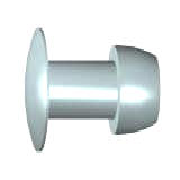
# Autodesk Inventor part: IFI 114 - .125  x .36
Saved by Autodesk Inventor 2012 (Build 160160000, 160)
## iProperties
Created: 2011-02-07
Part Number: IFI 114 - .125  x .36
Material: Steel, Mild
Description: Regular Protruding Head Style Break Mandrel Blind Rivet - Inch
Document SubType Name: Modeling
Standard: IFI 114
Designer: t_walti
Standard Revision: 2003
Standards Organization: ANSI
Language: en-US
Size Designation: 66
Categories: <MemberInstance><Categories><Category DisplayName="Fasteners" InternalName="e4da775c-781d-43d5-af7c-5136215cf5a6" Mnemonic="FSTN"><Category DisplayName="Rivets" InternalName="cf3d8c00-4198-4f00-854b-0d52b0adb238" Mnemonic="RIVET"><CategoryParameter DisplayName="Nominal Diameter" InternalName="0b221833-a430-4b2f-a4d4-a4e7cdbab5fe" Mnemonic="nomdia"/><CategoryParameter DisplayName="Nominal Length" InternalName="184b63f4-60b5-4ddb-b59d-a876aedee7db" Mnemonic="nomlen"/><CategoryParameter DisplayName="Functional Length" InternalName="2e4ddd0b-69f7-4d63-b45a-ef59153ff940" Mnemonic="fnclen"/><CategoryParameter DisplayName="Type" InternalName="841ce55c-7089-4646-bdbb-4888c77f269c" Mnemonic="type"/><CategoryParameter DisplayName="Grip Range (Min.-Max.)" InternalName="b095e0a4-6026-43f1-9b5f-1a93f7499cb0" Mnemonic="grprng"/><Category DisplayName="Plain" InternalName="0955f08f-2c95-4108-bac3-e7e722525866" Mnemonic="PLNRIVET"/></Category></Category><Category DisplayName="DataType" InternalName="23b78d0f-2648-40c6-8793-ca6db495c9e8" Mnemonic="DATATYPE"><CategoryParameter DisplayName="DisplayName" InternalName="05415f3d-3907-474b-a020-eb9d644f4cf3" Mnemonic="DISPLAYNAME"/><CategoryParameter DisplayName="InternalName" InternalName="cf1d0246-76d9-4b4a-8305-fa0409afb5c1" Mnemonic="INTERNALNAME"/><CategoryParameter DisplayName="Folder Name" InternalName="3f06958e-8713-4116-9be7-ed6184ecc97b" Mnemonic="FOLDERNAME"/><CategoryParameter DisplayName="Family Version" InternalName="914462f6-6e19-4b14-ba84-155b9680b1d0" Mnemonic="FAMILYREVISION"/><CategoryParameter DisplayName="ClipFormat" InternalName="bc51e27b-3422-4e78-93ef-cec197ddf230" Mnemonic="CLIPFORMAT"/><CategoryParameter DisplayName="IsMetric" InternalName="e2385c5b-1ea4-4823-96a8-8de651266ec3" Mnemonic="ISMETRIC"/><CategoryParameter DisplayName="Description" InternalName="13903e3d-64b1-4950-80da-f627842ea37f" Mnemonic="DESCRIPTION"/><CategoryParameter DisplayName="StdsOrg" InternalName="8f5914e1-4693-403f-8ab5-d37768198c9d" Mnemonic="STDSORG"/><CategoryParameter DisplayName="Standard" InternalName="0c0a119c-1e12-4c84-803f-101930972f5e" Mnemonic="STANDARD"/><CategoryParameter DisplayName="Manufacturer" InternalName="cd6c7a72-a28a-4e50-99a9-2c7f4e13e5ad" Mnemonic="MANUFACTURER"/><CategoryParameter DisplayName="Member Revision" InternalName="a65d44b9-392f-4f4f-857b-e4b3d54996fe" Mnemonic="MEMBERREVISION"/><CategoryParameter DisplayName="Standard Revision" InternalName="91d5a463-65c2-4fde-b823-3b7fea5e8e17" Mnemonic="STANDARDREVISION"/><CategoryParameter DisplayName="Revision Guid" InternalName="45a75005-10b1-4dfc-8d6d-dfe629f0b93c" Mnemonic="REVISIONGUID"/><CategoryParameter DisplayName="Designation" InternalName="2675968c-4ce5-49e0-a4f5-552d29089031" Mnemonic="DESIGNATION"/><CategoryParameter DisplayName="FileName" InternalName="8b46a4cc-9585-4fed-90c3-899f57e09a73" Mnemonic="FILENAME"/><CategoryParameter DisplayName="Default Row" InternalName="2af9ec52-faaa-4026-b378-f9fa4afca842" Mnemonic="DEFAULTROW"/><Category DisplayName="Part" InternalName="c0e0b642-3bcb-4cc8-9e80-f96d35c4afa4" Mnemonic="PART"><CategoryParameter DisplayName="Material" InternalName="818a152a-d3c3-49ca-80ee-df7d91421b8e" Mnemonic="MATERIAL"/><CategoryParameter DisplayName="Material Key" InternalName="5c9a8adb-dd2b-4535-b97f-0a94a95fe41f" Mnemonic="MATERIALKEY"/><CategoryParameter DisplayName="Part Number" InternalName="016b6077-bfbe-49bd-92c9-d8d59c39c941" Mnemonic="PARTNUMBER"/><CategoryParameter DisplayName="Stock Number" InternalName="4dba7c1c-e26c-444e-836c-b08b433409a8" Mnemonic="STOCKNUMBER"/></Category></Category><Category DisplayName="LegacyMap" InternalName="cd87c42b-3e48-431e-b5c0-1cbeb14dfe77" Mnemonic="LEGACYMAP"><CategoryParameter DisplayName="CatalogName" InternalName="d99d1e27-aa94-4de2-af4c-c348882a6f4f" Mnemonic="CATALOGNAME"/><CategoryParameter DisplayName="FamilyNumber" InternalName="e705e1f4-09cb-413e-91f9-551b4188271e" Mnemonic="FAMILYNUMBER"/><CategoryParameter DisplayName="MemberID" InternalName="8e5e0294-fc51-4c8f-b3d7-003dc5ed94f6" Mnemonic="MEMBERID"/><CategoryParameter DisplayName="unique CC member ID" InternalName="5193edd4-b2b0-4ab4-9d54-de900eee34e0" Mnemonic="CCCOOKIE"/><CategoryParameter DisplayName="unique DA member ID" InternalName="0918ad47-427f-4fed-ae26-24c81c58f590" Mnemonic="DACOOKIE"/><CategoryParameter DisplayName="Merge11 ID" InternalName="0ee8fb18-e2ed-4f39-96f6-1f4b5f50aa71" Mnemonic="MERGE11"/><CategoryParameter DisplayName="Split ID" InternalName="72b5c83c-be7f-45c4-ae51-9160ea6deb26" Mnemonic="SPLIT"/></Category></Categories><FamilyTemplate Id="ri0001"><FamilyTemplateParameters><FamilyTemplateParameter ObjectType="kUserParameterObject" ValueType="xs:double" Id="1" ObjectReferenceKey="R1"/><FamilyTemplateParameter ObjectType="kUserParameterObject" ValueType="xs:double" Id="2" ObjectReferenceKey="KOD"/><FamilyTemplateParameter ObjectType="kUserParameterObject" ValueType="xs:double" Id="3" ObjectReferenceKey="BOR"/><FamilyTemplateParameter ObjectType="kUserParameterObject" ValueType="xs:double" Id="4" ObjectReferenceKey="PHH"/><FamilyTemplateParameter ObjectType="kUserParameterObject" ValueType="xs:double" Id="5" ObjectReferenceKey="NND"/><FamilyTemplateParameter ObjectType="kUserParameterObject" ValueType="xs:double" Id="6" ObjectReferenceKey="KLG"/><FamilyTemplateParameter ObjectType="kUserParameterObject" ValueType="xs:double" Id="7" ObjectReferenceKey="KLGMAX"/><FamilyTemplateParameter ObjectType="kUserParameterObject" ValueType="xs:double" Id="8" ObjectReferenceKey="KOH"/><FamilyTemplateParameter ObjectType="kUserParameterObject" ValueType="xs:double" Id="9" ObjectReferenceKey="KLGMIN"/><FamilyTemplateParameter ObjectType="kPropertyObject" ValueType="xs:string" Id="100" ObjectReferenceKey="{32853F0F-3444-11d1-9E93-0060B03C1CA6}" SubObjectId="52"/><FamilyTemplateParameter ObjectType="kPropertyObject" ValueType="xs:string" Id="105" ObjectReferenceKey="{32853F0F-3444-11d1-9E93-0060B03C1CA6}" SubObjectId="5"/><FamilyTemplateParameter ObjectType="kPartComponentDefinitionObject" ValueType="xs:string" Id="110" SubObjectId="Material"/></FamilyTemplateParameters></FamilyTemplate><CategoryParameterMap><ParamToTemplateMap><ParamToTemplate CategoryParameter="//CategoryParameter[@InternalName='05415f3d-3907-474b-a020-eb9d644f4cf3']" ConstantValue="Regular Protruding Head Style Break Mandrel Blind Rivet (Inch) (IFI)"/><ParamToTemplate CategoryParameter="//CategoryParameter[@InternalName='cf1d0246-76d9-4b4a-8305-fa0409afb5c1']" ConstantValue="b007ff4d-50a3-4cbc-aa5a-b75e20d450cd"/><ParamToTemplate CategoryParameter="//CategoryParameter[@InternalName='3f06958e-8713-4116-9be7-ed6184ecc97b']" ConstantValue="IFI 114(4)"/><ParamToTemplate CategoryParameter="//CategoryParameter[@InternalName='914462f6-6e19-4b14-ba84-155b9680b1d0']" ConstantValue="10"/><ParamToTemplate CategoryParameter="//CategoryParameter[@InternalName='bc51e27b-3422-4e78-93ef-cec197ddf230']" ConstantValue="CF_INVENTOR.STDPARTS"/><ParamToTemplate CategoryParameter="//CategoryParameter[@InternalName='e2385c5b-1ea4-4823-96a8-8de651266ec3']" ConstantValue="false"/><ParamToTemplate CategoryParameter="//CategoryParameter[@InternalName='13903e3d-64b1-4950-80da-f627842ea37f']" ConstantValue="Regular Protruding Head Style Break Mandrel Blind Rivet - Inch"/><ParamToTemplate CategoryParameter="//CategoryParameter[@InternalName='8f5914e1-4693-403f-8ab5-d37768198c9d']" ConstantValue="ANSI"/><ParamToTemplate CategoryParameter="//CategoryParameter[@InternalName='0c0a119c-1e12-4c84-803f-101930972f5e']" ConstantValue="IFI 114"/><ParamToTemplate CategoryParameter="//CategoryParameter[@InternalName='cd6c7a72-a28a-4e50-99a9-2c7f4e13e5ad']" TemplateParameter="104"/><ParamToTemplate CategoryParameter="//CategoryParameter[@InternalName='91d5a463-65c2-4fde-b823-3b7fea5e8e17']" ConstantValue="2003"/><ParamToTemplate CategoryParameter="//CategoryParameter[@InternalName='45a75005-10b1-4dfc-8d6d-dfe629f0b93c']" ConstantValue="92a414c9-0dfd-4a8a-86e0-b3adb112cc1b"/><ParamToTemplate CategoryParameter="//CategoryParameter[@InternalName='2af9ec52-faaa-4026-b378-f9fa4afca842']" ConstantValue="10"/><ParamToTemplate CategoryParameter="//CategoryParameter[@InternalName='d99d1e27-aa94-4de2-af4c-c348882a6f4f']" ConstantValue="ANSI"/><ParamToTemplate CategoryParameter="//CategoryParameter[@InternalName='e705e1f4-09cb-413e-91f9-551b4188271e']" ConstantValue="1123"/><ParamToTemplate CategoryParameter="//CategoryParameter[@InternalName='8b46a4cc-9585-4fed-90c3-899f57e09a73']" ConstantValue="IFI 114 - 66 x .36(4)"/><ParamToTemplate CategoryParameter="//CategoryParameter[@InternalName='a65d44b9-392f-4f4f-857b-e4b3d54996fe']" ConstantValue="c1e365bb-b061-42a6-b7ff-1cacd618005e"/><ParamToTemplate CategoryParameter="//CategoryParameter[@InternalName='184b63f4-60b5-4ddb-b59d-a876aedee7db']" ConstantValue="0.575"/><ParamToTemplate CategoryParameter="//CategoryParameter[@InternalName='b095e0a4-6026-43f1-9b5f-1a93f7499cb0']" ConstantValue="0.251 - 0.375"/><ParamToTemplate CategoryParameter="//CategoryParameter[@InternalName='8e5e0294-fc51-4c8f-b3d7-003dc5ed94f6']" ConstantValue="210"/><ParamToTemplate CategoryParameter="//CategoryParameter[@InternalName='2675968c-4ce5-49e0-a4f5-552d29089031']" TemplateParameter="100"/><ParamToTemplate CategoryParameter="//CategoryParameter[@InternalName='2e4ddd0b-69f7-4d63-b45a-ef59153ff940']" TemplateParameter="6"/><ParamToTemplate CategoryParameter="//CategoryParameter[@InternalName='818a152a-d3c3-49ca-80ee-df7d91421b8e']" TemplateParameter="110"/><ParamToTemplate CategoryParameter="//CategoryParameter[@InternalName='0b221833-a430-4b2f-a4d4-a4e7cdbab5fe']" TemplateParameter="5"/><ParamToTemplate CategoryParameter="//CategoryParameter[@InternalName='016b6077-bfbe-49bd-92c9-d8d59c39c941']" TemplateParameter="105"/></ParamToTemplateMap></CategoryParameterMap></MemberInstance>
Density: 7.86 g/cm^3
Mass: 1.48656 g
Surface Area: 2.5312 cm^2
Volume: 0.18913 cm^3
IsCustomPart: 1
Author: t_walti
Autodesk Inventor part; units mm, degrees
ref_plane "YZ Plane" through (0, 0, 0) normal (1, 0, 0) x (0, 1, 0)
ref_plane "XZ Plane" through (0, 0, 0) normal (0, 1, 0) x (-1, 0, 0)
ref_plane "XY Plane" through (0, 0, 0) normal (0, 0, 1) x (1, 0, 0)
sketch "Sketch1" plane through (0, 0, 0) normal (0, 0, 1) x (1, 0, 0)
  line L0 (-0.2794, 3.3401) -> (0, 3.3401)
  line L1 (0, 3.3401) -> (0, 1.5875)
  line L2 (0, 1.5875) -> (9.145, 1.5875)
  line L3 (9.145, 1.5875) -> (9.145, 2.4049)
  line L4 (-1.524, 0) -> (13.717, 0)
  arc A0 (-0.2794, 3.3401) -> (-1.524, 0) centre (3.5802, 0) ccw
  line L5 (13.717, 0) -> (13.717, 1.8371)
  arc A1 (13.717, 1.8371) -> (9.145, 2.4049) centre (10.6582, -4.1017) ccw
  line L6 (-4.95, 0) -> (16.8866, 0) projected
  line L7 (0, -8.6865) -> (0, 7.3745) projected
  dimension "d0" = 6.6802
  dimension "d1" = 3.175
  dimension "d2" = 4.8097
  dimension "d3" = 3.6741
  dimension "d4" = 6.6802
  dimension "d5" = 4.572
  dimension "d6" = 9.145
  dimension "d7" = 0.2794
  dimension "d8" = 1.524
  constraints: 12 end point, 4 point on circle, 3 perpendicular, 2 centre point, 2 collinear, 2 parallel, 1 horizontal, 1 point on line
  measures "d0" diameter of L0 L4
  measures "d1" diameter of L2 L4
  measures "d2" diameter of L3.end L4
  measures "d3" diameter of L5.end L4
  measures "d4" radius of A1
  measures "d5" distance between parallel lines of L5 L3
  measures "d6" distance of L1.end L2.end
  measures "d7" distance of L0.start L0.end
  measures "d8" distance from line of L4.start L1
revolve "Body" add sketch "Sketch1" angle 360 about axis through (-1.524, 0, 0) along (1, 0, 0)
fillet "Fillet1" radius 0.635 1 edges at (0, -1.5875, 0)
equation "\"d10\" = R1"
equation "\"d0\" = KOD"
equation "\"d1\" = NND"
equation "\"d2\" = 0.72 * KOD"
equation "\"d3\" = 0.55 * KOD"
equation "\"d4\" = KOD"
equation "\"d5\" = 3 * KOH"
equation "\"d7\" = PHH"
equation "\"d8\" = KOH"
equation "\"NND\" = 3.175"
equation "\"KLG\" = 9.144"
equation "\"KOH\" = 1.524"
equation "\"KOD\" = 6.6802"
equation "\"PHH\" = 0.2794"
equation "\"R1\" = 0.635"
equation "\"BOR\" = 2.8956"
equation "\"KLGMAX\" = 9.525"
equation "\"KLGMIN\" = 6.3754"
body "Solid1"
